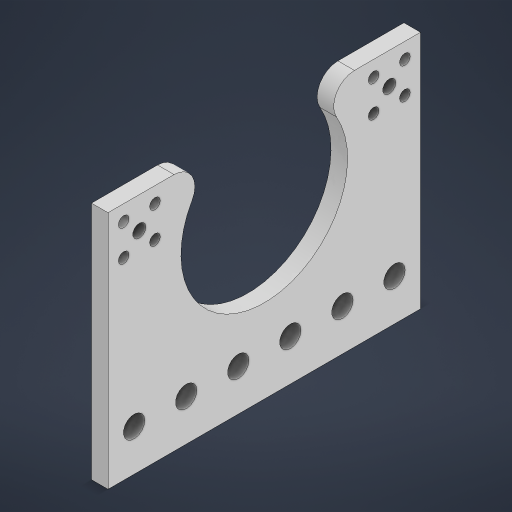
# Autodesk Inventor part: FirstStageMotorSupportPlate
Saved by Autodesk Inventor 2024 (Build 280153000, 153)
## iProperties
Created: 2024-01-05
Part Number: FirstStageMotorSupportPlate
Material: Generic
Document SubType Name: Modeling
Designer: avsar
Density: 1 g/cm^3
Appearance: Default
Author: avsar
Autodesk Inventor part; units mm, degrees
ref_plane "YZ Plane" through (0, 0, 0) normal (1, 0, 0) x (0, 1, 0)
ref_plane "XZ Plane" through (0, 0, 0) normal (0, 1, 0) x (-1, 0, 0)
ref_plane "XY Plane" through (0, 0, 0) normal (0, 0, 1) x (1, 0, 0)
sketch "Sketch1" plane through (0, 0, 0) normal (1, 0, 0) x (0, 1, 0)
  line L0 (-46, 60) -> (46, 60)
  line L1 (46, 60) -> (46, -60)
  line L2 (46, -60) -> (-46, -60)
  line L3 (-46, -60) -> (-46, 60)
  line L4 (-46, 60) -> (46, -60) construction
  line L5 (46, 60) -> (-46, -60) construction
  point P0 (0, 0)
  dimension "d0" = 92
  dimension "d1" = 120
  constraints: 12 end point, 2 midpoint, 2 parallel, 1 horizontal, 1 perpendicular
  measures "d0" distance of L1.end L2.end
  measures "d1" distance of L0.end L1.end
extrude "Extrusion1" add sketch "Sketch1" along normal blind 6.35
sketch "Sketch2" plane through (6.35, 0, 0) normal (1, 0, 0) x (0, 0, -1)
  circle A0 centre (-50, -30.125) radius 4.1
  line L0 (-60, -46) -> (60, -46) construction
  circle A1 centre (-30, -30.125) radius 4.1
  circle A2 centre (-10, -30.125) radius 4.1
  circle A3 centre (10, -30.125) radius 4.1
  circle A4 centre (30, -30.125) radius 4.1
  circle A5 centre (50, -30.125) radius 4.1
  point P0 (0, 0)
  dimension "d4" = 8.2
  dimension "d5" = 15.875
  dimension "d6" = 50
  dimension "d9" = 20
  constraints: 6 centre point, 1 horizontal, 10 other
  measures "d4" diameter of A0
  measures "d5" distance from line of L0 A0.centre
  measures "d6" horizontal distance of point (0, 0) A0.centre
  measures "d9" distance of A0.centre A1.centre
extrude "Extrusion2" cut sketch "Sketch2" against normal through all
sketch "Sketch3" plane through (6.35, 0, 0) normal (1, 0, 0) x (0, 0, -1)
  circle A0 centre (0, 18) radius 32
  line L0 (-60, -46) -> (60, -46) projected
  point P0 (0, 0)
  point P1 (0, -46)
  dimension "d16" = 64
  dimension "d17" = 64
  constraints: 1 centre point, 1 midpoint, 1 vertical alignment
  measures "d16" diameter of A0
  measures "d17" distance of point (0, -46) A0.centre
extrude "Extrusion3" cut sketch "Sketch3" against normal through all
fillet "Fillet1" radius 8 2 edges at (3.175, 46, -15.4919) (3.175, 46, 15.4919)
sketch "Sketch4" plane through (6.35, 0, 0) normal (1, 0, 0) x (0, 0, -1)
  circle A0 centre (-48, 34) radius 2.5
  circle A1 centre (-54, 40) radius 2.05
  circle A2 centre (-54, 28) radius 2.05
  circle A3 centre (-42, 28) radius 2.05
  circle A4 centre (-42, 40) radius 2.05
  line L0 (-60, 46) -> (-60, -46) construction
  line L1 (-34.641, 46) -> (-60, 46) construction
  line L2 (0, 0) -> (0, -14) construction
  arc A5 (-27.7128, 34) -> (27.7128, 34) centre (0, 18) ccw construction
  circle A6 centre (48, 34) radius 2.5
  circle A7 centre (54, 40) radius 2.05
  circle A8 centre (54, 28) radius 2.05
  circle A9 centre (42, 28) radius 2.05
  circle A10 centre (42, 40) radius 2.05
  dimension "d23" = 5
  dimension "d24" = 4.1
  dimension "d25" = 6
  dimension "d26" = 6
  dimension "d29" = 360
  dimension "d31" = 12
  dimension "d32" = 12
  constraints: 10 centre point, 5 symmetric about line, 2 end point, 1 point on circle, 1 vertical, 14 other
  measures "d23" diameter of A0
  measures "d24" diameter of A1
  measures "d25" horizontal distance of A1.centre A0.centre
  measures "d26" horizontal distance of A0.centre A1.centre
  measures "d31" distance from line of L0 A0.centre
  measures "d32" distance from line of L1 A0.centre
extrude "Extrusion4" cut sketch "Sketch4" against normal through all
body "Solid1"
